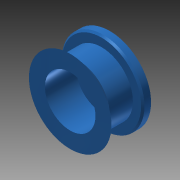
# Autodesk Inventor part: pully 15mmx25mmx12mm
Saved by Autodesk Inventor 2013 SP2 (Build 170200200, 200)
## iProperties
Created: 2016-11-25
Part Number: pully 15mmx25mmx12mm
Material: Generic
Document SubType Name: Modeling
Designer: hdv
Density: 1 g/cm^3
Mass: 2.16109 g
Surface Area: 23.9465 cm^2
Volume: 2.16109 cm^3
Author: hdv
Autodesk Inventor part; units mm, degrees
ref_plane "YZ Plane" through (0, 0, 0) normal (1, 0, 0) x (0, 1, 0)
ref_plane "XZ Plane" through (0, 0, 0) normal (0, 1, 0) x (-1, 0, 0)
ref_plane "XY Plane" through (0, 0, 0) normal (0, 0, 1) x (1, 0, 0)
sketch "Sketch1" plane through (0, 0, 0) normal (0, 0, 1) x (1, 0, 0)
  line L0 (7.65, 0) -> (12.5, 0)
  line L1 (12.5, 0) -> (12.5, 12) construction
  line L2 (12.5, 12) -> (7.65, 12)
  line L3 (7.65, 12) -> (7.65, 0)
  line L4 (0, 0) -> (0, 8.5122) construction
  line L5 (9.5, 9.5) -> (9.5, 2.5)
  line L6 (9.5, 9.5) -> (12, 9.5)
  line L7 (12, 9.5) -> (12.5, 10)
  line L8 (12.5, 0) -> (9.5, 2.5)
  line L9 (12.5, 10) -> (12.5, 12)
  line L10 (7.65, 12) -> (5.65, 12)
  line L11 (5.65, 12) -> (5.65, 9.5)
  line L12 (5.65, 9.5) -> (7.65, 9.5)
  line L13 (7.65, 9.5) -> (7.65, 12)
  point P0 (12.5, 0.6699)
  point P1 (12.5, 6)
  point P2 (15.2143, 7.5754)
  point P3 (15.2143, 2.4246)
  point P4 (9.5, 6)
  point P5 (17.7886, 0.302)
  point P6 (7.65, 6)
  dimension "d6" = 12
  dimension "d7" = 7.65
  dimension "d17" = 7
  dimension "d18" = 2.5
  dimension "d19" = 135
  dimension "d20" = 3
  dimension "d21" = 2
  dimension "d22" = 2.5
  dimension "d23" = 12.5
  constraints: 28 end point, 4 parallel, 3 midpoint, 3 perpendicular, 2 horizontal, 2 horizontal alignment, 2 point on line, 2 vertical, 1 coincident, 1 collinear
  measures "d6" distance of L1.end L0.end
  measures "d7" distance from line of L3 point (0, 0)
  measures "d17" distance of L5.start L5.end
  measures "d18" distance of L5.start L6.end
  measures "d19" angle of L7 L6
  measures "d20" distance between parallel lines of L1 L5
  measures "d21" distance of L12.end L11.end
  measures "d22" distance of L11.end L10.end
  measures "d23" distance of L0.end point (0, 0)
revolve "Revolution1" add sketch "Sketch1" angle 360 about axis through (0, 0, 0) along (0, 1, 0)
body "Solid1"
